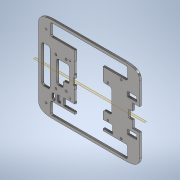
# Autodesk Inventor part: CAT_protector
Saved by Autodesk Inventor 2022 (Build 260153000, 153)
## iProperties
Created: 2024-07-28
Part Number: CAT_protector
Material: Типовые
Document SubType Name: Sheet Metal
Designer: Капустяник Андрей
Density: 1 g/cm^3
Sheet Metal Rule: По умолчанию
Appearance: Сталь — полированная
Author: Капустяник Андрей
Autodesk Inventor part; units mm, degrees
(part 1 of 2)
ref_plane "YZ Plane" through (0, 0, 0) normal (1, 0, 0) x (0, 1, 0)
ref_plane "XZ Plane" through (0, 0, 0) normal (0, 1, 0) x (-1, 0, 0)
ref_plane "XY Plane" through (0, 0, 0) normal (0, 0, 1) x (1, 0, 0)
sketch "Эскиз1" plane through (0, 0, 0) normal (0, 0, 1) x (1, 0, 0)
  line L0 (73, -60.7947) -> (73, -48.7947)
  line L1 (-3, -60.7947) -> (-73, -60.7947)
  line L2 (75, -60.7227) -> (75, -58.3095)
  line L3 (6, -60.7947) -> (70, -60.7947)
  spline S0 degree 4 poles (55, -66.7947) (62.0326, -66.7947) (73.0217, -66.3174) (75, -62.6206) (75, -58.3095) knots 0 0 0 0 0 1 1 1 1 1
  spline S1 degree 2 poles (-55, -66.7947) (-75.0547, -67.2536) (-75, -58.3095) knots 0 0 0 1 1 1
  spline S2 degree 2 poles (55, 66.7947) (75.0195, 66.261) (75, 58.3095) knots 0 0 0 1 1 1
  spline S3 degree 2 poles (-55, 66.7947) (-75.2212, 66.9636) (-75, 58.3095) knots 0 0 0 1 1 1
  line L4 (-60.2698, -62.7947) -> (55, -62.7947)
  line L5 (60, -58.3095) -> (60, -62.7947)
  line L6 (60, -62.7947) -> (55, -62.7947)
  line L7 (60, 62.7947) -> (-60, 62.7947)
  line L8 (55, 66.7947) -> (-55, 66.7947)
  line L9 (-75, 58.3095) -> (-75, -58.3095)
  line L10 (55, -66.7947) -> (-55, -66.7947)
  line L11 (75, -58.3095) -> (75, 58.3095)
  line L12 (60, -62.7947) -> (-60, -62.7947)
  line L13 (-60, 62.7947) -> (60, 62.7947)
  line L14 (-75, 40.5) -> (-75, 43.5)
  line L15 (75, 40.5) -> (75, 43.5)
  line L16 (75, -40.5) -> (75, -43.5)
  line L17 (-75, -40.5) -> (-75, -43.5)
  line L18 (-75, -40.5) -> (-75, -43.5)
  line L19 (75, -40.5) -> (75, -43.5)
  line L20 (-60, -40.5) -> (60, -40.5)
  line L21 (60, -43.5) -> (-60, -43.5)
  line L22 (-60, 43.5) -> (60, 43.5)
  line L23 (60, 40.5) -> (-60, 40.5)
  line L24 (0, -43.5) -> (4, -43.5)
  line L25 (4, -43.5) -> (4, -62.7947)
  line L26 (4, -43.5) -> (-4, -43.5)
  line L27 (-4, -43.5) -> (-4, -62.7947)
  line L28 (0, 43.5) -> (4, 43.5)
  line L29 (4, 43.5) -> (4, 62.7947)
  line L30 (4, 62.7947) -> (-4, 62.7947)
  line L31 (-4, 62.7947) -> (-4, 43.5)
  line L32 (-60, 43.5) -> (60, 43.5)
  line L33 (60, 40.5) -> (-60, 40.5)
  line L34 (-60, -43.5) -> (60, -43.5)
  line L35 (60, -40.5) -> (-60, -40.5)
  line L36 (-60, -62.7947) -> (-60, -43.5)
  line L37 (-60, -40.5) -> (-60, 40.5)
  line L38 (-60, 62.7947) -> (-60, 43.5)
  line L39 (60, 62.7947) -> (60, 43.5)
  line L40 (60, 40.5) -> (60, -40.5)
  line L41 (60, -43.5) -> (60, -58.3095)
  line L42 (60, 43.5) -> (60, -43.5)
  line L43 (-60, 43.5) -> (-60, -43.5)
  line L44 (-55, 66.7947) -> (-55, 64.6653)
  line L45 (-55, 64.6653) -> (-63.94, 64.6653)
  line L46 (-63.94, 64.6653) -> (-63.94, 58.3095)
  line L47 (-63.94, 58.3095) -> (-75, 58.3095)
  line L48 (-55, -66.7947) -> (-55, -64.5292)
  line L49 (-55, -64.5292) -> (-62.0706, -64.5292)
  line L50 (-62.0706, -64.5292) -> (-62.0706, -58.3095)
  line L51 (-62.0706, -58.3095) -> (-75, -58.3095)
  line L52 (55, -66.7947) -> (55, -65.0318)
  line L53 (55, -65.0318) -> (61.8678, -65.0318)
  line L54 (61.8678, -65.0318) -> (61.8678, -58.3095)
  line L55 (61.8678, -58.3095) -> (75, -58.3095)
  line L56 (55, 66.7947) -> (55, 64.6653)
  line L57 (55, 64.6653) -> (61.3837, 64.6653)
  line L58 (61.3837, 64.6653) -> (61.3837, 58.3095)
  line L59 (61.3837, 58.3095) -> (75, 58.3095)
  point P0 (-73, -48.7947)
  point P1 (72.3235, -63.7587)
  point P2 (-72.3272, -63.6113)
  point P3 (72.5326, 62.9869)
  point P4 (-72.4994, 63.4051)
  dimension "d14" = 4
  dimension "d15" = 8
  dimension "d16" = 4
  dimension "d17" = 8
  measures "d14" distance of L24.start L24.end
  measures "d15" distance of L24.end L26.end
  measures "d16" distance of L28.start L28.end
  measures "d17" distance of L29.end L30.end
extrude "Пластина2" add sketch "Эскиз1" along normal blind 3 contours L36 L4 L6 L5 L3 L54 L53 L52 L10 L48 L49 L50 L1 | L1 L50 L51 L9 L47 L46 L45 L44 L8 L56 L57 L58 L59 L11 L55 L54 L3 L5 L41 L42 L40 L39 L7 L38 L43 L37 L36 | L37 L23 L40 L20
sketch "Эскиз2" plane through (0, 0, 3) normal (0, 0, 1) x (1, 0, 0)
  line L0 (-75, 58.3095) -> (-75, -58.3095)
  line L1 (-75, 0) -> (-79, 0)
  line L2 (75, -58.3095) -> (75, 58.3095)
  line L3 (75, 0) -> (79, 0)
  line L4 (-79, 52.7636) -> (-79, -52.7636)
  line L5 (79, 52.7636) -> (79, -52.7636)
  line L6 (-60, 62.7947) -> (60, 62.7947)
  line L7 (60, -62.7947) -> (-60, -62.7947)
  line L8 (-75, -58.3095) -> (-75, 58.3095)
  line L9 (55, -66.7947) -> (-55, -66.7947)
  line L10 (75, 58.3095) -> (75, -58.3095)
  line L11 (-55, 66.7947) -> (55, 66.7947)
  line L12 (-55, -66.7947) -> (55, -66.7947)
  line L13 (-55, -66.7947) -> (-55, -63.9796)
  line L14 (-55, -63.9796) -> (-61.4162, -63.9796)
  line L15 (-61.4162, -63.9796) -> (-61.4162, 0)
  line L16 (-61.4162, 0) -> (-79, 0)
  line L17 (55, 66.7947) -> (-55, 66.7947)
  line L18 (-55, 66.7947) -> (-55, 63.9478)
  line L19 (-55, 63.9478) -> (-61.4162, 63.9478)
  line L20 (-61.4162, 63.9478) -> (-61.4162, 0)
  line L21 (-79, 0) -> (-61.4162, 0)
  line L22 (60, 62.7947) -> (-60, 62.7947)
  line L23 (-75, -58.3095) -> (-75, 58.3095)
  line L24 (-75, 58.3095) -> (-75, 62.3095)
  line L25 (-75, -58.3095) -> (-75, -62.3095)
  spline S0 degree 4 poles (-79, -52.7636) (-79, -59.2344) (-76.8822, -65.8429) (-63.8717, -66.7947) (-55, -66.7947) knots 0 0 0 0 0 1 1 1 1 1
  line L26 (-60, 40.5) -> (-60, 62.7947)
  line L27 (60, 62.7947) -> (60, 40.5)
  line L28 (-60, 40.5) -> (60, 40.5)
  line L29 (61.3837, 58.3095) -> (75, 58.3095)
  line L30 (61.3837, 64.6653) -> (61.3837, 58.3095)
  line L31 (55, 64.6653) -> (61.3837, 64.6653)
  line L32 (55, 66.7947) -> (55, 64.6653)
  line L33 (-55, 64.6653) -> (-55, 66.7947)
  line L34 (-63.94, 64.6653) -> (-55, 64.6653)
  line L35 (-63.94, 58.3095) -> (-63.94, 64.6653)
  line L36 (-75, 58.3095) -> (-63.94, 58.3095)
  line L37 (-62.0706, -58.3095) -> (-75, -58.3095)
  line L38 (-62.0706, -64.5292) -> (-62.0706, -58.3095)
  line L39 (-55, -64.5292) -> (-62.0706, -64.5292)
  line L40 (-55, -66.7947) -> (-55, -64.5292)
  line L41 (55, -65.0318) -> (55, -66.7947)
  line L42 (61.8678, -65.0318) -> (55, -65.0318)
  line L43 (61.8678, -58.3095) -> (61.8678, -65.0318)
  line L44 (75, -58.3095) -> (61.8678, -58.3095)
  line L45 (60, -40.5) -> (-60, -40.5)
  line L46 (60, -40.5) -> (60, -62.7947)
  line L47 (-60, -62.7947) -> (-60, -40.5)
  spline S1 degree 4 poles (-55, 66.7947) (-63.8717, 66.7947) (-76.8822, 65.8429) (-79, 59.2344) (-79, 52.7636) knots 0 0 0 0 0 1 1 1 1 1
  line L48 (-55, 66.7947) -> (55, 66.7947)
  line L49 (55, -66.7947) -> (-55, -66.7947)
  line L50 (75, -58.3095) -> (75, -62.3095)
  line L51 (75, 58.3095) -> (75, 62.3095)
  line L52 (-55, 66.7947) -> (0, 66.7947)
  line L53 (0, 66.7947) -> (55, 66.7947)
  spline S2 degree 4 poles (55, -66.7947) (63.8717, -66.7947) (76.8822, -65.8429) (79, -59.2344) (79, -52.7636) knots 0 0 0 0 0 1 1 1 1 1
  line L54 (55, 64.6653) -> (55, 66.7947)
  spline S3 degree 4 poles (55, 66.7947) (63.8717, 66.7947) (76.8822, 65.8429) (79, 59.2344) (79, 52.7636) knots 0 0 0 0 0 1 1 1 1 1
  line L55 (55, -66.7947) -> (55, -65.0318)
  line L56 (55, -65.0318) -> (60.9248, -65.0318)
  line L57 (60.9248, -65.0318) -> (60.9248, 64.6653)
  line L58 (61.3837, 64.6653) -> (55, 64.6653)
  line L59 (55, 64.6653) -> (55, 66.7947)
  line L60 (55, 64.6653) -> (60.9248, 64.6653)
  line L61 (61.8678, -65.0318) -> (55, -65.0318)
  point P0 (0, 0)
  dimension "d18" = 4
  dimension "d19" = 4
  dimension "d121" = 4
  dimension "d122" = 4
  dimension "d123" = 4
  dimension "d124" = 4
  dimension "d125" = 55
  measures "d18" distance of L1.end L1.start
  measures "d19" distance of L3.end L3.start
  measures "d121" distance of L0.start L24.end
  measures "d122" distance of L8.start L25.end
  measures "d123" distance of L10.end L50.end
  measures "d124" distance of L10.start L51.end
  measures "d125" distance of L52.end L11.end
sheet face with bend "Грань4" sketch "Эскиз2" thickness 3 toward (0, 0, -1) bend radius 3 contours L0 L1 L4 S1 L24 | L24 S1 L18 L34 L35 L36 | L0 L25 S0 L4 L1 | L37 L38 L39 L13 S0 L25 | S3 L51 L29 L30 L31 L32 | L41 L42 L43 L44 L50 S2 | S3 L5 L3 L2 L51 | L50 L2 L3 L5 S2
bend "Сгиб2"
sketch "Эскиз3" plane through (0, 0, 3) normal (0, 0, 1) x (1, 0, 0)
  line L0 (-79, 40.5) -> (-21.945, 40.5) projected
  line L1 (-62.1467, -40.5) -> (-79, -40.5) projected
  line L2 (-55, 66.7947) -> (55, 66.7947) projected
  line L3 (55, -66.7947) -> (-55, -66.7947) projected
  line L4 (60, 62.7947) -> (60, 40.5) projected
  line L5 (60, -62.7947) -> (-60, -62.7947) projected
  line L6 (-60, 40.5) -> (-60, 62.7947) projected
  line L7 (-60, 62.7947) -> (60, 62.7947) projected
  line L8 (68, -17.5) -> (79, -17.5)
  line L9 (79, -17.5) -> (79, 17.5)
  line L10 (79, 17.5) -> (68, 17.5)
  line L11 (68, 17.5) -> (68, -17.5)
  line L12 (-68, -17.5) -> (-79, -17.5) projected
  line L13 (-79, -17.5) -> (-79, -40.5) projected
  line L14 (-62.1467, -40.5) -> (-62.1467, -10.5) projected
  line L15 (-62.1467, -10.5) -> (-36.1467, -10.5) projected
  line L16 (-36.1467, -10.5) -> (-36.1467, -40.5) projected
  line L17 (-21.945, -40.5) -> (-21.945, 40.5) projected
  line L18 (-79, 40.5) -> (-79, 17.5) projected
  line L19 (-79, 17.5) -> (-68, 17.5) projected
  line L20 (-68, 17.5) -> (-68, -17.5) projected
  line L21 (-21.945, -40.5) -> (-36.1467, -40.5) projected
  line L22 (79, -5) -> (68, -5)
  line L23 (68, -5) -> (68, 5)
  line L24 (68, 5) -> (79, 5)
  line L25 (79, 5) -> (79, -5)
  line L26 (79, -5) -> (68, 5) construction
  line L27 (68, -5) -> (79, 5) construction
  line L28 (79, 52.7636) -> (79, 0) projected
  ellipse E0 centre (78.3753, -19.3) end of major axis (79, -19.3) minor radius 0.5 (78.3753, -19.8) -> (79, -19.3) ccw projected
  line L29 (79, -19.3) -> (79, -17.5) projected
  line L30 (79, -17.5) -> (68, -17.5) projected
  line L31 (68, -17.5) -> (68, -6) projected
  line L32 (68, -6) -> (63.1467, -6) projected
  arc A0 (62.1467, -5) -> (63.1467, -6) centre (63.1467, -5) ccw projected
  line L33 (62.1467, -5) -> (62.1467, 5) projected
  arc A1 (63.1467, 6) -> (62.1467, 5) centre (63.1467, 5) ccw projected
  line L34 (63.1467, 6) -> (68, 6) projected
  line L35 (68, 6) -> (68, 17.5) projected
  line L36 (68, 17.5) -> (79, 17.5) projected
  line L37 (79, 17.5) -> (79, 19.3) projected
  ellipse E1 centre (78.3753, 19.3) end of major axis (79, 19.3) minor radius 0.5 (79, 19.3) -> (78.3753, 19.8) ccw projected
  line L38 (78.3753, 19.8) -> (62.1467, 19.8) projected
  line L39 (62.1467, 19.8) -> (62.1467, 10.5) projected
  line L40 (62.1467, 10.5) -> (36.1467, 10.5) projected
  line L41 (36.1467, 10.5) -> (36.1467, 40.5) projected
  line L42 (21.945, 40.5) -> (36.1467, 40.5) projected
  line L43 (21.945, 40.5) -> (21.945, -40.5) projected
  line L44 (62.1467, -40.5) -> (21.945, -40.5) projected
  line L45 (62.1467, -40.5) -> (62.1467, -19.8) projected
  line L46 (62.1467, -19.8) -> (78.3753, -19.8) projected
  line L47 (68, -6) -> (79, -6)
  line L48 (68, 6) -> (79, 6)
  line L49 (60, -40.5) -> (-60, -40.5) projected
  line L50 (60, -40.5) -> (60, -62.7947) projected
  line L51 (-60, -62.7947) -> (-60, -40.5) projected
  line L52 (-60, 40.5) -> (60, 40.5) projected
  line L53 (-79, 52.7636) -> (-79, -52.7636) projected
  line L54 (79, -52.7636) -> (79, 52.7636) projected
  line L55 (79, -6) -> (63.1467, -6)
  line L56 (63.1467, 6) -> (79, 6)
  line L57 (79, 6) -> (79, -6)
  line L58 (68, -17.5) -> (79, -17.5)
  line L59 (79, -17.5) -> (79, 17.5)
  line L60 (79, 17.5) -> (68, 17.5)
  line L61 (68, 17.5) -> (68, -17.5)
  point P0 (0, 0)
  point P1 (79, -52.7636)
  point P2 (73.5, 0)
  dimension "d54" = 10
  constraints: 38 end point, 7 parallel, 4 collinear, 4 perpendicular, 3 horizontal, 3 point on line, 2 midpoint, 10 other
  measures "d54" distance of L22.end L23.end
extrude "Вырез1" cut sketch "Эскиз3" against normal blind 3 contours L8 L11 L47 L9 | L9 L48 L11 L10 | L47 L11 L22 L9 | L9 L24 L11 L48 | L32 A0 L33 A1 L34 L11 | L22 L11 L24 L9
sketch "Эскиз5" plane through (0, 0, 3) normal (0, 0, 1) x (1, 0, 0)
  line L0 (65.1786, -28.7) -> (72.0893, -28.7) projected
  line L1 (72.0893, -22.5) -> (65.1786, -22.5) projected
  line L2 (72.0893, 22.5) -> (65.1786, 22.5) projected
  line L3 (65.1786, 28.7) -> (72.0893, 28.7) projected
  line L4 (61.2, 28.5) -> (74.1, 28.5)
  line L5 (74.1, 28.5) -> (74.1, 22.7)
  line L6 (74.1, 22.7) -> (61.2, 22.7)
  line L7 (61.2, 22.7) -> (61.2, 28.5)
  line L8 (61.2, -22.7) -> (74.1, -22.7)
  line L9 (74.1, -22.7) -> (74.1, -28.5)
  line L10 (74.1, -28.5) -> (61.2, -28.5)
  line L11 (61.2, -28.5) -> (61.2, -22.7)
  line L12 (60.4, -21.9) -> (74.9, -21.9)
  line L13 (74.9, -21.9) -> (74.9, -29.3)
  line L14 (74.9, -29.3) -> (60.4, -29.3)
  line L15 (60.4, -29.3) -> (60.4, -21.9)
  line L16 (74.9, 29.3) -> (60.4, 29.3)
  line L17 (60.4, 29.3) -> (60.4, 21.9)
  line L18 (60.4, 21.9) -> (74.9, 21.9)
  line L19 (74.9, 21.9) -> (74.9, 29.3)
  point P0 (0, 0)
  point P1 (61.35, -39.5)
  point P2 (74.1, -27.9)
  point P3 (61.2, -22.1)
  point P4 (79, -52.7636)
  dimension "d133" = 0.8
  dimension "d134" = 0.8
  constraints: 32 end point, 8 parallel, 4 perpendicular, 2 horizontal, 13 other
  measures "d133" distance between parallel lines of L11 L15
  measures "d134" distance between parallel lines of L4 L16
extrude "Вырез3" cut sketch "Эскиз5" against normal blind 3 contours L4 L5 L6 L7 | L8 L9 L10 L11 | L12 L13 L14 L15 | L19 L18 L17 L16
sketch "Эскиз6" plane through (0, 0, 3) normal (0, 0, 1) x (1, 0, 0)
  line L0 (-22.0704, -43.5) -> (-22.0704, -28.4138)
  line L1 (-22.0704, -43.5) -> (-39.0704, -43.5)
  line L2 (-39.0704, -28.4138) -> (-39.0704, -43.5)
  line L3 (-22.0704, -28.4138) -> (-39.0704, -28.4138)
  line L4 (-60, 62.7947) -> (-60, -62.7947)
  line L5 (-22.0704, -43.5) -> (-60, -43.5)
  line L6 (-60, -43.5) -> (-60, -28.4138)
  line L7 (-60, -28.4138) -> (-22.0704, -28.4138)
  line L8 (-22.0704, -28.4138) -> (-22.0704, -43.5)
  line L9 (-22.0704, 43.5) -> (-60, 43.5)
  line L10 (-60, 43.5) -> (-60, 28.4138)
  line L11 (-60, 28.4138) -> (-22.0704, 28.4138)
  line L12 (-22.0704, 28.4138) -> (-22.0704, 43.5)
  line L13 (74.5523, 43.5) -> (-79, 43.5)
  line L14 (-68, 0) -> (-60, 0)
  line L15 (-60, 28.4138) -> (-22.0704, 28.4138)
  line L16 (-22.0704, 28.4138) -> (-32.0704, 28.4138)
  line L17 (-32.0704, 28.4138) -> (-32.0704, -28.4138)
  line L18 (-32.0704, -28.4138) -> (-22.0704, -28.4138)
  line L19 (-22.0704, -28.4138) -> (-22.0704, 28.4138)
  line L20 (-32.0704, 28.4138) -> (-60, 28.4138)
  line L21 (-60, 28.4138) -> (-60, 23.4138)
  line L22 (-60, 23.4138) -> (-32.0704, 23.4138)
  line L23 (-32.0704, 23.4138) -> (-32.0704, 28.4138)
  line L24 (-32.0704, -28.4138) -> (-60, -28.4138)
  line L25 (-60, -28.4138) -> (-60, -23.4138)
  line L26 (-60, -23.4138) -> (-32.0704, -23.4138)
  line L27 (-32.0704, -23.4138) -> (-32.0704, -28.4138)
  line L28 (-60, 23.4138) -> (-60, -23.4138)
  point P0 (0, 0)
  dimension "d45" = 10
  dimension "d52" = 5
  dimension "d53" = 5
  measures "d45" distance between parallel lines of L17 L19
  measures "d52" distance between parallel lines of L11 L22
  measures "d53" distance between parallel lines of L7 L26
sheet face with bend "Грань5" sketch "Эскиз6" thickness 3 toward (0, 0, -1) bend radius 3
bend "Сгиб3"
sketch "Эскиз7" plane through (0, 0, 3) normal (0, 0, 1) x (1, 0, 0)
  line L0 (55, -66.7947) -> (-55, -66.7947)
  line L1 (-55, 66.7947) -> (55, 66.7947)
  line L2 (-60, 43.5) -> (-60, 62.7947)
  line L3 (-60, 62.7947) -> (60, 62.7947)
  line L4 (60, 62.7947) -> (60, 40.5)
  line L5 (60, -62.7947) -> (-60, -62.7947)
  line L6 (-60, -62.7947) -> (-60, -43.5)
  spline S0 degree 4 poles (-74.5618, -40.5) (-74.5618, -41.2011) (-74.563, -41.9466) (-74.5609, -42.7177) (-74.5523, -43.5) knots 0 0 0 0 0 1 1 1 1 1
  line L7 (-74.5523, -43.5) -> (79, -43.5)
  line L8 (79, -40.5) -> (79, -43.5)
  line L9 (79, -40.5) -> (-74.5618, -40.5)
  spline S1 degree 4 poles (74.5618, 40.5) (74.5618, 41.2011) (74.563, 41.9466) (74.5609, 42.7177) (74.5523, 43.5) knots 0 0 0 0 0 1 1 1 1 1
  line L10 (74.5523, 43.5) -> (-79, 43.5)
  line L11 (-79, 40.5) -> (-79, 43.5)
  line L12 (-79, 40.5) -> (74.5618, 40.5)
  line L13 (60, -62.7947) -> (60, 62.7947)
  line L14 (60, 43.5) -> (56.75, 43.5)
  line L15 (56.75, 43.5) -> (56.75, -43.5)
  line L16 (56.75, -43.5) -> (60, -43.5)
  line L17 (60, -43.5) -> (60, 43.5)
  arc A0 (62.1467, -5) -> (63.1467, -6) centre (63.1467, -5) ccw
  line L18 (62.1467, -5) -> (62.1467, 5)
  arc A1 (63.1467, 6) -> (62.1467, 5) centre (63.1467, 5) ccw
  line L19 (-60, -43.5) -> (-22.0704, -43.5)
  line L20 (-22.0704, -43.5) -> (-22.0704, -40.5)
  line L21 (-22.0704, 43.5) -> (-60, 43.5)
  line L22 (-22.0704, 40.5) -> (60, 40.5)
  line L23 (-22.0704, 40.5) -> (-22.0704, 43.5)
  line L24 (60, -40.5) -> (-22.0704, -40.5)
  line L25 (60, -40.5) -> (60, -62.7947)
  line L26 (-79, 52.7636) -> (-79, -52.7636)
  line L27 (79, -52.7636) -> (79, -17.5)
  line L28 (79, 17.5) -> (79, 52.7636)
  line L29 (63.1467, 6) -> (68, 6)
  line L30 (68, 6) -> (68, 17.5)
  line L31 (68, 17.5) -> (79, 17.5)
  line L32 (79, -17.5) -> (68, -17.5)
  line L33 (68, -17.5) -> (68, -6)
  line L34 (68, -6) -> (63.1467, -6)
  point P0 (0, 0)
  constraints: 8 end point, 3 point on line, 2 parallel, 1 horizontal, 1 perpendicular, 8 other
sheet face with bend "Грань6" sketch "Эскиз7" thickness 3 toward (0, 0, -1) bend radius 3 contours L10 L4 L12 L15 | L12 L13 L9 L15 | L9 L13 L7 L15
bend "Сгиб4"
sketch "Эскиз8" plane through (0, 0, 3) normal (0, 0, 1) x (1, 0, 0)
  line L0 (-29.7061, 17.7) -> (-45.6809, 17.7)
  line L1 (-29.7061, -5.8) -> (-44.2713, -5.8)
  ellipse E0 centre (-48.9698, 13.2) end of major axis (-48.9698, 16.7) minor radius 1.1971 projected
  line L2 (-29.7061, 17.7) -> (-33.7061, 17.7)
  line L3 (-48.9698, 13.2) -> (-48.9698, -5.8)
  line L4 (-48.9698, -5.8) -> (-44.2713, -5.8)
  line L5 (-33.7061, 17.7) -> (-48.9698, 17.7)
  line L6 (-48.9698, 17.7) -> (-48.9698, -5.8)
  line L7 (-48.9698, -5.8) -> (-33.7061, -5.8)
  line L8 (-33.7061, -5.8) -> (-33.7061, 17.7)
  line L9 (-30.7061, 20.7) -> (-30.7061, -8.8)
  line L10 (-30.7061, -8.8) -> (-51.9698, -8.8)
  line L11 (-51.9698, -8.8) -> (-51.9698, 20.7)
  line L12 (-51.9698, 20.7) -> (-30.7061, 20.7)
  line L13 (-32.7061, 18.7) -> (-49.9698, 18.7)
  line L14 (-49.9698, 18.7) -> (-49.9698, -6.8)
  line L15 (-49.9698, -6.8) -> (-32.7061, -6.8)
  line L16 (-32.7061, -6.8) -> (-32.7061, 18.7)
  line L17 (-32.7061, 18.7) -> (-30.7061, 18.7)
  line L18 (-32.7061, -6.8) -> (-30.7061, -6.8)
  line L19 (-49.9698, 18.7) -> (-50.4698, 18.7)
  line L20 (-50.4698, 18.7) -> (-50.4698, -6.8)
  line L21 (-50.4698, -6.8) -> (-49.9698, -6.8)
  line L22 (-49.9698, -6.8) -> (-49.9698, 18.7)
  point P0 (0, 0)
  dimension "d55" = 4
  dimension "d56" = 3
  dimension "d57" = 3
  dimension "d60" = 2
  dimension "d96" = 0.5
  constraints: 46 end point, 7 perpendicular, 4 horizontal, 4 parallel, 3 point on line, 1 collinear, 1 vertical, 9 other
  measures "d55" distance of L0.start L2.end
  measures "d56" distance between parallel lines of L8 L9
  measures "d57" distance between parallel lines of L6 L11
  measures "d60" distance between parallel lines of L12 L13
  measures "d96" distance of L21.end L20.end
extrude "Вырез4" cut sketch "Эскиз8" against normal blind 3 contours L8 L1 L4 L3 E0 L6 L5 L0 | L0 L5 L6 E0 L14 L13 L16 | L0 L16 L1 L8 | L16 L17 L9 L0 | L0 L9 L1 L16 | L1 L16 L15 L14 E0 L3 L4 | L1 L9 L18 L16 | L6 L3 E0 L14 | E0 L3 L6 | L14 E0 L21 L20 L19 | L14 E0
sketch "Эскиз9" plane through (0, 0, 3) normal (0, 0, 1) x (1, 0, 0)
  line L0 (-60, 5) -> (-60, -5) projected
  line L1 (-60, 5) -> (-22.0704, 5)
  line L2 (-22.0704, 5) -> (-22.0704, -5)
  line L3 (-22.0704, -5) -> (-60, -5)
  line L4 (-60, -5) -> (-60, 5)
  line L5 (-60, -5) -> (-79, -5) projected
  line L6 (-22.0704, -5) -> (-25.0704, -5)
  line L7 (-25.0704, -5) -> (-25.0704, 5)
  line L8 (-25.0704, 5) -> (-22.0704, 5)
  line L9 (-22.0704, 5) -> (-22.0704, -5)
  line L10 (-27.1601, 11.2623) -> (-27.1601, -11.2623) projected
  line L11 (-22.0704, -43.5) -> (-22.0704, 43.5) projected
  line L12 (-22.8704, 9.6299) -> (-22.8704, 25.277) projected
  line L13 (-22.8704, -9.6299) -> (-22.8704, -25.277) projected
  line L14 (-23.1963, -10.238) -> (-23.1963, -27.6138) projected
  line L15 (-23.1963, -10.238) -> (-23.1963, -27.6138) projected
  line L16 (-23.1963, -27.6138) -> (-27.1633, -27.6138) projected
  line L17 (-23.1963, -27.6138) -> (-22.0704, -27.6138)
  line L18 (-22.0704, -27.6138) -> (-22.0704, -15.6138)
  line L19 (-22.0704, -15.6138) -> (-23.1963, -15.6138)
  line L20 (-23.1963, -15.6138) -> (-23.1963, -27.6138)
  line L21 (-23.1963, -10.238) -> (-22.0704, -10.238)
  line L22 (-22.0704, -10.238) -> (-22.0704, -22.238)
  line L23 (-22.0704, -22.238) -> (-23.1963, -22.238)
  line L24 (-23.1963, -22.238) -> (-23.1963, -10.238)
  line L25 (-23.1963, -27.6138) -> (-23.6963, -27.6138)
  line L26 (-23.6963, -27.6138) -> (-23.6963, -15.6138)
  line L27 (-23.6963, -15.6138) -> (-23.1963, -15.6138)
  line L28 (-23.1963, -15.6138) -> (-23.1963, -27.6138)
  line L29 (-23.1963, -10.238) -> (-23.6963, -10.238)
  line L30 (-23.6963, -10.238) -> (-23.6963, -22.238)
  line L31 (-23.6963, -22.238) -> (-23.1963, -22.238)
  line L32 (-23.1963, -22.238) -> (-23.1963, -10.238)
  ellipse E0 centre (-16.5786, 0) end of major axis (-16.5786, -50) minor radius 17.101 (-33.3998, 9.0085) -> (-33.3998, -9.0085) ccw projected
  ellipse E1 centre (-29.7061, 0) end of major axis (-29.7061, 13.5) minor radius 4.6173 (-27.1601, 11.2623) -> (-33.2518, 8.6474) ccw projected
  ellipse E2 centre (-29.7061, 0) end of major axis (-29.7061, 13.5) minor radius 4.6173 (-33.2518, -8.6474) -> (-27.1601, -11.2623) ccw projected
  line L33 (-33.2518, -8.6474) -> (-33.3998, -9.0085) projected
  line L34 (-33.3998, 9.0085) -> (-33.2518, 8.6474) projected
  line L35 (-22.0704, 0) -> (-23.4463, 0)
  line L36 (-23.1963, 10.238) -> (-23.1963, 27.6138)
  line L37 (-23.1963, 27.6138) -> (-22.0704, 27.6138)
  line L38 (-23.1963, 10.238) -> (-22.0704, 10.238)
  line L39 (-23.1963, 10.238) -> (-22.0704, 10.238)
  line L40 (-22.0704, 10.238) -> (-22.0704, 27.6138)
  line L41 (-22.0704, 27.6138) -> (-23.1963, 27.6138)
  line L42 (-23.1963, 27.6138) -> (-23.1963, 10.238)
  point P0 (0, 0)
  point P1 (-75, -5)
  dimension "d61" = 3
  dimension "d71" = 12
  dimension "d72" = 12
  dimension "d73" = 0.5
  constraints: 64 end point, 14 parallel, 8 horizontal, 7 perpendicular, 5 collinear, 5 symmetric about line, 3 point on line, 1 midpoint, 3 other
  measures "d61" distance of L7.end L8.end
  measures "d71" distance of L18.end L17.end
  measures "d72" distance of L21.end L22.end
  measures "d73" distance of L26.end L27.end
extrude "Вырез5" cut sketch "Эскиз9" against normal blind 3 contours L1 L2 L3 L7 | L17 L14 L23 L11 | L23 L13 L19 L11 | L19 L13 L21 L11 | L23 L14 L19 L13 | L19 L14 L21 L13 | L38 L36 L37 L11
sketch "Эскиз10" plane through (0, 0, 3) normal (0, 0, 1) x (1, 0, 0)
  line L0 (-22.0704, -35.8733) -> (-22.0704, -66.7947)
  line L1 (-19.85, -40.5) -> (74, -40.5)
  line L2 (74, 40.5) -> (-19.85, 40.5)
  line L3 (56.75, 43.5) -> (56.75, -43.5)
  line L4 (-22.0704, -43.5) -> (-22.0704, 43.5)
  line L5 (56.75, 43.5) -> (-22.0704, 43.5)
  line L6 (-22.0704, 43.5) -> (-22.0704, 40.5)
  line L7 (-22.0704, 40.5) -> (56.75, 40.5)
  line L8 (56.75, 40.5) -> (56.75, 43.5)
  line L9 (60, -43.5) -> (60, -62.7947)
  line L10 (-22.0704, -43.5) -> (-22.0704, 43.5)
  line L11 (60, -43.5) -> (-22.0704, -43.5)
  line L12 (-22.0704, -43.5) -> (-22.0704, -40.5)
  line L13 (-22.0704, -40.5) -> (60, -40.5)
  line L14 (60, -40.5) -> (60, -43.5)
  point P0 (0, 0)
  point P1 (-21.95, 40.5)
  point P2 (-22.0704, 5)
  point P3 (-22.0704, -5)
sheet face with bend "Грань7" sketch "Эскиз10" thickness 3 toward (0, 0, -1) bend radius 3 contours L13 L1 L3 L11 L0 | L4 L5 L3 L2 L7 | L3 L1 L14 L11
bend "Сгиб5"
sketch "Эскиз11" plane through (0, 0, 0) normal (0, 0, -1) x (-1, 0, 0)
  circle A0 centre (51.6714, 23.0046) radius 2.1 projected
  circle A1 centre (51.6714, -23.0046) radius 2.1 projected
  circle A2 centre (31.1704, 33.954) radius 2.1 projected
  circle A3 centre (31.1704, -33.954) radius 2.1 projected
  circle A4 centre (31.1704, -33.954) radius 2.1 projected
  circle A5 centre (31.1704, 33.954) radius 2.1 projected
  circle A6 centre (31.1704, -33.954) radius 1.5
  circle A7 centre (31.1704, 33.954) radius 1.5
  circle A8 centre (51.6714, 23.0046) radius 1.5
  circle A9 centre (51.6714, -23.0046) radius 1.5
  circle A10 centre (31.1704, -33.954) radius 2.1 projected
  line L0 (78.7, 7.7813) -> (41.2823, 7.7813) projected
  circle A11 centre (31.1704, 33.954) radius 2.1 projected
  point P0 (0, 0)
  dimension "d88" = 3
  dimension "d89" = 3
  dimension "d90" = 3
  dimension "d91" = 3
  constraints: 4 centre point, 4 coincident
  measures "d88" diameter of A6
  measures "d89" diameter of A7
  measures "d90" diameter of A8
  measures "d91" diameter of A9
extrude "Вырез6" cut sketch "Эскиз11" against normal blind 3 contours A8 | A9
fillet "Сопряжение1" radius 3 4 edges at (-30.7061, 18.7, 1.5) (-30.7061, -6.8, 1.5) (-50.4698, 18.7, 1.5) (-50.4698, -6.8, 1.5)
sketch "Эскиз13" plane through (0, 0, 3) normal (0, 0, 1) x (1, 0, 0)
  line L0 (60, 43.5) -> (-60, 43.5) projected
  line L1 (-60, 43.5) -> (-60, 62.7947) projected
  line L2 (-60, 62.7947) -> (60, 62.7947) projected
  line L3 (60, 62.7947) -> (60, 43.5) projected
  line L4 (-60, -43.5) -> (60, -43.5) projected
  line L5 (60, -43.5) -> (60, -62.7947) projected
  line L6 (60, -62.7947) -> (-60, -62.7947) projected
  line L7 (-60, -62.7947) -> (-60, -43.5) projected
  line L8 (55, -66.7947) -> (-55, -66.7947) projected
  arc A0 (62.1467, -5) -> (63.1467, -6) centre (63.1467, -5) ccw projected
  line L9 (62.1467, -5) -> (62.1467, 5) projected
  arc A1 (63.1467, 6) -> (62.1467, 5) centre (63.1467, 5) ccw projected
  line L10 (-55, 66.7947) -> (55, 66.7947) projected
  line L11 (-47.4698, 18.7) -> (-33.7061, 18.7) projected
  arc A2 (-30.7061, 15.7) -> (-33.7061, 18.7) centre (-33.7061, 15.7) ccw projected
  line L12 (-30.7061, 15.7) -> (-30.7061, -3.8) projected
  arc A3 (-33.7061, -6.8) -> (-30.7061, -3.8) centre (-33.7061, -3.8) ccw projected
  line L13 (-33.7061, -6.8) -> (-47.4698, -6.8) projected
  line L14 (-22.0704, -27.6138) -> (-23.1963, -27.6138) projected
  line L15 (-23.1963, -27.6138) -> (-23.1963, -10.238) projected
  line L16 (-23.1963, -10.238) -> (-22.0704, -10.238) projected
  line L17 (-22.0704, -5) -> (-25.0704, -5) projected
  line L18 (-25.0704, -5) -> (-25.0704, 5) projected
  line L19 (-25.0704, 5) -> (-22.0704, 5) projected
  line L20 (-22.0704, 10.238) -> (-23.1963, 10.238) projected
  line L21 (-23.1963, 10.238) -> (-23.1963, 27.6138) projected
  line L22 (-23.1963, 27.6138) -> (-22.0704, 27.6138) projected
  line L23 (-60, -43.5) -> (60, -43.5) projected
  line L24 (60, 43.5) -> (-60, 43.5) projected
  line L25 (21.945, -43.5) -> (-22.0704, -43.5)
  line L26 (-22.0704, 43.5) -> (21.945, 43.5)
  line L27 (21.945, 43.5) -> (21.945, -43.5)
  line L28 (21.945, 40.5) -> (21.945, -40.5) projected
  line L29 (-22.0704, -43.5) -> (-23.0704, -43.5)
  line L30 (-22.0704, 43.5) -> (-23.0704, 43.5)
  line L31 (-50.4698, -3.8) -> (-50.4698, 15.7) projected
  arc A4 (-47.4698, 18.7) -> (-50.4698, 15.7) centre (-47.4698, 15.7) ccw projected
  arc A5 (-50.4698, -3.8) -> (-47.4698, -6.8) centre (-47.4698, -3.8) ccw projected
  line L32 (-22.0704, 5) -> (-22.0704, -5) projected
  line L33 (-22.0704, -10.238) -> (-22.0704, -27.6138) projected
  line L34 (-22.0704, 27.6138) -> (-22.0704, 10.238) projected
  line L35 (-79, 52.7636) -> (-79, -52.7636) projected
  line L36 (79, -52.7636) -> (79, -17.5) projected
  line L37 (79, 17.5) -> (79, 52.7636) projected
  line L38 (63.1467, 6) -> (68, 6) projected
  line L39 (-21, -40.5) -> (-21, -43.5) projected
  line L40 (21, -43.5) -> (21, -40.5) projected
  line L41 (-18, 40.5) -> (-21, 40.5) projected
  line L42 (-21, 43.5) -> (-21, 40.5) projected
  line L43 (21, 40.5) -> (21, 43.5) projected
  line L44 (21, 43.5) -> (21, -43.5)
  line L45 (-60, -43.5) -> (60, -43.5) projected
  line L46 (21, 40.5) -> (21, 43.5) projected
  line L47 (-21, 43.5) -> (-21, 40.5) projected
  line L48 (-21, 43.5) -> (-22.0704, 43.5)
  line L49 (-22.0704, 43.5) -> (-22.0704, 40)
  line L50 (-21, -43.5) -> (-22.0704, -43.5)
  line L51 (-22.0704, -43.5) -> (-22.0704, -40)
  line L52 (-22.0704, -43.5) -> (-22.0704, 43.5)
  line L53 (60, 43.5) -> (-60, 43.5) projected
  line L54 (-22.0704, 40) -> (-23.0704, 40)
  line L55 (-23.0704, 40) -> (-23.0704, 43.5)
  line L56 (-23.0704, 43.5) -> (-22.0704, 43.5)
  line L57 (-22.0704, 43.5) -> (-22.0704, 40)
  line L58 (-22.0704, -40) -> (-23.0704, -40)
  line L59 (-23.0704, -40) -> (-23.0704, -43.5)
  line L60 (-23.0704, -43.5) -> (-22.0704, -43.5)
  line L61 (-22.0704, -43.5) -> (-22.0704, -40)
  line L62 (-22.0704, 27.6138) -> (-22.0704, 10.238) projected
  line L63 (21.945, -43.5) -> (-22.0704, -43.5)
  line L64 (-22.0704, -43.5) -> (-22.0704, 43.5)
  line L65 (-22.0704, 43.5) -> (21.945, 43.5)
  line L66 (21.945, 43.5) -> (21.945, -43.5)
  line L67 (68, 6) -> (68, 17.5) projected
  line L68 (68, 17.5) -> (79, 17.5) projected
  line L69 (79, -17.5) -> (68, -17.5) projected
  line L70 (68, -17.5) -> (68, -6) projected
  line L71 (68, -6) -> (63.1467, -6) projected
  point P0 (0, 0)
  dimension "d127" = 3.5
  dimension "d129" = 3.5
  dimension "d130" = 1
  dimension "d131" = 1
  constraints: 46 end point, 8 horizontal, 7 parallel, 5 perpendicular, 2 collinear, 2 point on line, 1 vertical, 13 other
  measures "d127" distance of L49.end L48.end
  measures "d129" distance of L50.end L51.end
  measures "d130" distance of L55.end L56.end
  measures "d131" distance of L60.end L59.end
extrude "Вырез7" cut sketch "Эскиз13" against normal blind 3 contours L27 L4 L40 L44 L43 L0 | L43 L44 L40 L4 L51 L52 L33 L32 L34 L49 L0
sketch "Эскиз14" plane through (0, 0, 3) normal (0, 0, 1) x (1, 0, 0)
  circle A0 centre (29.5, -25.5) radius 1.6 projected
  circle A1 centre (29.5, 25.5) radius 1.6 projected
  circle A2 centre (-29.5, 25.5) radius 1.6 projected
  circle A3 centre (-29.5, 25.5) radius 1.25
  circle A4 centre (29.5, 25.5) radius 1.25
  circle A5 centre (29.5, -25.5) radius 1.25
  circle A6 centre (-29.5, -25.5) radius 1.6 projected
  circle A7 centre (-29.5, -25.5) radius 1.25
  point P0 (-31.1704, -33.954)
  dimension "d106" = 2.5
  dimension "d107" = 2.5
  dimension "d108" = 2.5
  dimension "d110" = 2.5
  constraints: 4 centre point, 4 coincident
  measures "d106" diameter of A3
  measures "d107" diameter of A4
  measures "d108" diameter of A5
  measures "d110" diameter of A7
extrude "Вырез8" cut sketch "Эскиз14" against normal blind 3 contours A3 | A4 | A5 | A7
sketch "Эскиз18" plane through (0, 0, 3) normal (0, 0, 1) x (1, 0, 0)
  line L0 (36.945, -29.6) -> (36.945, -39.6)
  line L1 (21.945, -29.6) -> (36.945, -29.6)
  line L2 (36.945, -39.6) -> (31.5198, -39.6)
  line L3 (-50.4698, -3.8) -> (-50.4698, 15.7)
  arc A0 (-47.4698, 18.7) -> (-50.4698, 15.7) centre (-47.4698, 15.7) ccw
  line L4 (-47.4698, 18.7) -> (-33.7061, 18.7)
  arc A1 (-30.7061, 15.7) -> (-33.7061, 18.7) centre (-33.7061, 15.7) ccw
  line L5 (-30.7061, 15.7) -> (-30.7061, -3.8)
  arc A2 (-33.7061, -6.8) -> (-30.7061, -3.8) centre (-33.7061, -3.8) ccw
  line L6 (-33.7061, -6.8) -> (-47.4698, -6.8)
  arc A3 (-50.4698, -3.8) -> (-47.4698, -6.8) centre (-47.4698, -3.8) ccw
  circle A4 centre (-51.6714, -23.0046) radius 1.5
  circle A5 centre (-51.6714, 23.0046) radius 1.5
  line L7 (60, 43.5) -> (21.945, 43.5)
  line L8 (-60, 43.5) -> (-60, 62.7947)
  line L9 (-60, 62.7947) -> (60, 62.7947)
  line L10 (60, 62.7947) -> (60, 43.5)
  line L11 (60, -43.5) -> (60, -62.7947)
  line L12 (60, -62.7947) -> (-60, -62.7947)
  line L13 (-60, -62.7947) -> (-60, -43.5)
  line L14 (-22.0704, -27.6138) -> (-23.1963, -27.6138)
  line L15 (-23.1963, -27.6138) -> (-23.1963, -10.238)
  line L16 (-23.1963, -10.238) -> (-22.0704, -10.238)
  line L17 (-22.0704, -5) -> (-25.0704, -5)
  line L18 (-25.0704, -5) -> (-25.0704, 5)
  line L19 (-25.0704, 5) -> (-22.0704, 5)
  line L20 (-22.0704, 10.238) -> (-23.1963, 10.238)
  line L21 (-23.1963, 10.238) -> (-23.1963, 27.6138)
  line L22 (-23.1963, 27.6138) -> (-22.0704, 27.6138)
  circle A6 centre (-29.5, -25.5) radius 1.25
  circle A7 centre (29.5, 25.5) radius 1.25
  circle A8 centre (29.5, -25.5) radius 1.25
  circle A9 centre (-29.5, 25.5) radius 1.25
  line L23 (-55, 66.7947) -> (55, 66.7947)
  line L24 (55, -66.7947) -> (-55, -66.7947)
  arc A10 (62.1467, -5) -> (63.1467, -6) centre (63.1467, -5) ccw
  line L25 (62.1467, -5) -> (62.1467, 5)
  arc A11 (63.1467, 6) -> (62.1467, 5) centre (63.1467, 5) ccw
  line L26 (-22.7204, -40.6) -> (-39.6204, -40.6)
  line L27 (-23.7204, -29.6) -> (-37.9129, -29.6)
  line L28 (-22.7204, -29.6) -> (-39.6204, -29.6)
  line L29 (-39.6204, -29.6) -> (36.945, -29.6)
  line L30 (36.945, -39.6) -> (-39.6204, -39.6)
  line L31 (-39.6204, -39.6) -> (-39.6204, -40.6)
  line L32 (-39.6204, -40.6) -> (36.945, -40.6)
  line L33 (36.945, -40.6) -> (36.945, -39.6)
  line L34 (-39.6204, -29.6) -> (-39.6204, -39.6)
  line L35 (21.945, -29.6) -> (36.945, -29.6)
  line L36 (36.945, -29.6) -> (36.945, -28.1)
  line L37 (36.945, -28.1) -> (21.945, -28.1)
  line L38 (21.945, -28.1) -> (21.945, -29.6)
  line L39 (-79, 52.7636) -> (-79, -52.7636)
  line L40 (79, -52.7636) -> (79, -17.5)
  line L41 (79, 17.5) -> (79, 52.7636)
  line L42 (63.1467, 6) -> (68, 6)
  line L43 (-60, -43.5) -> (-22.0704, -43.5)
  line L44 (-22.0704, -10.238) -> (-22.0704, -5)
  line L45 (-22.0704, 5) -> (-22.0704, 10.238)
  line L46 (-22.0704, 27.6138) -> (-22.0704, 43.5)
  line L47 (-22.0704, 43.5) -> (-60, 43.5)
  line L48 (21.945, 43.5) -> (21.945, -43.5)
  line L49 (21.945, -43.5) -> (60, -43.5)
  line L50 (-22.0704, -43.5) -> (-22.0704, -27.6138)
  line L51 (68, 6) -> (68, 17.5)
  line L52 (68, 17.5) -> (79, 17.5)
  line L53 (79, -17.5) -> (68, -17.5)
  line L54 (68, -17.5) -> (68, -6)
  line L55 (68, -6) -> (63.1467, -6)
  point P0 (0, 0)
extrude "Вырез11" cut sketch "Эскиз18" against normal blind 3 contours L0 L2 L30 L48 L1 | L1 L38 L37 L36 | L33 L32 L48 L30 L2 | L48 L30 L50 L29 | L50 L30 L34 L28 L27 L29 | L48 L32 L50 L30 | L50 L32 L26 L31 L30
sketch "Эскиз19" plane through (0, 0, 3) normal (0, 0, 1) x (1, 0, 0)
  line L0 (32.4467, -6.7) -> (32.4467, 13.7)
  line L1 (32.4467, 13.7) -> (28.4467, 13.7)
  line L2 (28.4467, 13.7) -> (28.4467, -6.7)
  line L3 (28.4467, -6.7) -> (32.4467, -6.7)
  circle A0 centre (27.9467, 17.5) radius 1.6
  circle A1 centre (27.9467, -10.5) radius 1.6
  spline S0 degree 3 poles (63.6588, 29) (63.7235, 29) (63.7997, 29.0148) (63.9185, 29.063) (63.9826, 29.1046) (64.0726, 29.1925) (64.1149, 29.254) (64.1629, 29.3674) (64.1776, 29.439) (64.1776, 29.5) knots 0 0 0 0 0.25714 0.25714 0.510158 0.510158 0.757535 0.757535 1 1 1 1
  line L4 (60.1467, 29) -> (63.6588, 29)
  arc A2 (60.1467, 29) -> (59.1467, 28) centre (60.1467, 28) ccw
  line L5 (59.1467, 23.2) -> (59.1467, 28)
  arc A3 (59.1467, 23.2) -> (60.1467, 22.2) centre (60.1467, 23.2) ccw
  line L6 (67, 22.2) -> (60.1467, 22.2)
  arc A4 (68, 21.2) -> (67, 22.2) centre (67, 21.2) ccw
  line L7 (68, 6) -> (68, 21.2)
  line L8 (63.1467, 6) -> (68, 6)
  arc A5 (63.1467, 6) -> (62.1467, 5) centre (63.1467, 5) ccw
  line L9 (62.1467, -5) -> (62.1467, 5)
  arc A6 (62.1467, -5) -> (63.1467, -6) centre (63.1467, -5) ccw
  line L10 (68, -6) -> (63.1467, -6)
  line L11 (68, -14) -> (68, -6)
  line L12 (26.1467, -14) -> (68, -14)
  arc A7 (24.4467, -12.3) -> (26.1467, -14) centre (26.1467, -12.3) ccw
  line L13 (24.4467, 19.3) -> (24.4467, -12.3)
  arc A8 (26.1467, 21) -> (24.4467, 19.3) centre (26.1467, 19.3) ccw
  line L14 (34.1467, 21) -> (26.1467, 21)
  arc A9 (34.1467, 21) -> (36.4467, 23.3) centre (34.1467, 23.3) ccw
  line L15 (36.4467, 29.7) -> (36.4467, 23.3)
  arc A10 (36.4467, 29.7) -> (34.1467, 32) centre (34.1467, 29.7) ccw
  line L16 (32.1967, 32) -> (34.1467, 32)
  arc A11 (32.1967, 40.5) -> (32.1967, 32) centre (32.1967, 36.25) ccw
  line L17 (66.0967, 40.5) -> (32.1967, 40.5)
  arc A12 (66.0967, 32) -> (66.0967, 40.5) centre (66.0967, 36.25) ccw
  line L18 (64.6989, 32) -> (66.0967, 32)
  spline S1 degree 3 poles (64.1776, 31.5) (64.1776, 31.5609) (64.1923, 31.6325) (64.2403, 31.7458) (64.2825, 31.8072) (64.3726, 31.8952) (64.4369, 31.9368) (64.5566, 31.9852) (64.6336, 32) (64.6989, 32) knots 0 0 0 0 0.241518 0.241518 0.487947 0.487947 0.74085 0.74085 1 1 1 1
  line L19 (64.1776, 29.5) -> (64.1776, 31.5)
  circle A13 centre (66.0967, 36.25) radius 1.6
  circle A14 centre (32.1967, 36.25) radius 1.6
  line L20 (25.4467, 16.7) -> (35.4467, 16.7)
  line L21 (35.4467, 16.7) -> (35.4467, -9.7)
  line L22 (35.4467, -9.7) -> (25.4467, -9.7)
  line L23 (25.4467, -9.7) -> (25.4467, 16.7)
  circle A15 centre (27.9467, -10.5) radius 4.6
  circle A16 centre (27.9467, 17.5) radius 4.6
  line L24 (35.4467, -15.1) -> (21.945, -15.1)
  line L25 (21.945, -15.1) -> (21.945, 22.1)
  line L26 (21.945, 22.1) -> (35.4467, 22.1)
  line L27 (35.4467, 22.1) -> (35.4467, -15.1)
  line L28 (21.945, 43.5) -> (21.945, -28.1)
  point P0 (0, 0)
  dimension "d135" = 3
  dimension "d136" = 3
  dimension "d137" = 3
  constraints: 16 end point, 2 centre point, 2 collinear, 2 parallel, 2 tangent, 1 horizontal, 1 perpendicular, 3 other
  measures "d135" distance between parallel lines of L1 L20
  measures "d136" radial gap between concentric circles of A1 A15
  measures "d137" radial gap between concentric circles of A0 A16
extrude "Вырез12" cut sketch "Эскиз19" against normal blind 3 contours L3 A15 L2 A16 L1 L0 | L0 L1 A16 L20 L21 L22 A15 L3 | A15 L22 A1 L23 L2 L3 | L3 L2 A15 | A16 L2 L1 | L1 L2 A16 L23 L20 A0 | A15 L12 A7 L13 L23 L22 A1 | L22 L27 L12 A15 | A15 L23 A16 L2 | A16 L14 A9 L27 L20 | L20 A0 L23 A16 L13 A8 L14 | L22 A1 | A1 L22 | A15 L13 A16 L23 | L20 A0 | A0 L20 | L27 L24 A15 L12 | A15 L13 A7 L12 | A15 L24 L25 L26 A16 L13 | A16 L14 A8 L13 | A9 L14 A16 L26 L27
fillet "Сопряжение3" radius 3 4 edges at (35.4467, -15.1, 1.5) (21.945, -15.1, 1.5) (35.4467, 22.1, 1.5) (21.945, 22.1, 1.5)
fillet "Сопряжение4" radius 2 8 edges at (-60, -43.5, 1.5) (-60, -62.7947, 1.5) (60, -43.5, 1.5) (60, -62.7947, 1.5) (60, 62.7947, 1.5) (60, 43.5, 1.5) (-60, 62.7947, 1.5) (-60, 43.5, 1.5)
ref_plane "РабПлоскость1" through (63.1467, 0, 3) normal (0, 1, 0) x (1, 0, 0)
sketch "Эскиз20" plane through (0, 0, 0) normal (0, 0, -1) x (-1, 0, 0)
  arc A0 (-24.945, 22.1) -> (-21.945, 25.1) centre (-24.945, 25.1) ccw projected
  line L0 (-21.945, 25.1) -> (-21.945, 43.5) projected
  line L1 (-58, 43.5) -> (-21.945, 43.5) projected
  arc A1 (-60, 45.5) -> (-58, 43.5) centre (-58, 45.5) ccw projected
  line L2 (-60, 45.5) -> (-60, 60.7947) projected
  arc A2 (-58, 62.7947) -> (-60, 60.7947) centre (-58, 60.7947) ccw projected
  line L3 (-58, 62.7947) -> (58, 62.7947) projected
  arc A3 (60, 60.7947) -> (58, 62.7947) centre (58, 60.7947) ccw projected
  line L4 (60, 60.7947) -> (60, 45.5) projected
  arc A4 (58, 43.5) -> (60, 45.5) centre (58, 45.5) ccw projected
  line L5 (22.0704, 43.5) -> (58, 43.5) projected
  line L6 (22.0704, 43.5) -> (22.0704, 27.6138) projected
  line L7 (22.0704, 27.6138) -> (23.1963, 27.6138) projected
  line L8 (23.1963, 27.6138) -> (23.1963, 10.238) projected
  line L9 (23.1963, 10.238) -> (22.0704, 10.238) projected
  line L10 (22.0704, 10.238) -> (22.0704, 5) projected
  line L11 (22.0704, 5) -> (25.0704, 5) projected
  line L12 (25.0704, 5) -> (25.0704, -5) projected
  line L13 (25.0704, -5) -> (22.0704, -5) projected
  line L14 (22.0704, -5) -> (22.0704, -10.238) projected
  line L15 (22.0704, -10.238) -> (23.1963, -10.238) projected
  line L16 (23.1963, -10.238) -> (23.1963, -27.6138) projected
  line L17 (23.1963, -27.6138) -> (22.0704, -27.6138) projected
  line L18 (22.0704, -27.6138) -> (22.0704, -29.6) projected
  line L19 (22.0704, -29.6) -> (39.6204, -29.6) projected
  line L20 (39.6204, -29.6) -> (39.6204, -40.6) projected
  line L21 (39.6204, -40.6) -> (22.0704, -40.6) projected
  line L22 (22.0704, -40.6) -> (22.0704, -43.5) projected
  line L23 (58, -43.5) -> (22.0704, -43.5) projected
  arc A5 (60, -45.5) -> (58, -43.5) centre (58, -45.5) ccw projected
  line L24 (60, -45.5) -> (60, -60.7947) projected
  arc A6 (58, -62.7947) -> (60, -60.7947) centre (58, -60.7947) ccw projected
  line L25 (58, -62.7947) -> (-58, -62.7947) projected
  arc A7 (-60, -60.7947) -> (-58, -62.7947) centre (-58, -60.7947) ccw projected
  line L26 (-60, -60.7947) -> (-60, -45.5) projected
  arc A8 (-58, -43.5) -> (-60, -45.5) centre (-58, -45.5) ccw projected
  line L27 (-21.945, -43.5) -> (-58, -43.5) projected
  line L28 (-21.945, -43.5) -> (-21.945, -40.6) projected
  line L29 (-21.945, -40.6) -> (-36.945, -40.6) projected
  line L30 (-36.945, -40.6) -> (-36.945, -28.1) projected
  line L31 (-36.945, -28.1) -> (-21.945, -28.1) projected
  line L32 (-21.945, -28.1) -> (-21.945, -18.1) projected
  arc A9 (-21.945, -18.1) -> (-24.945, -15.1) centre (-24.945, -18.1) ccw projected
  line L33 (-24.945, -15.1) -> (-32.4467, -15.1) projected
  arc A10 (-35.4467, -12.1) -> (-32.4467, -15.1) centre (-32.4467, -12.1) ccw projected
  line L34 (-35.4467, -12.1) -> (-35.4467, 19.1) projected
  arc A11 (-32.4467, 22.1) -> (-35.4467, 19.1) centre (-32.4467, 19.1) ccw projected
  line L35 (-32.4467, 22.1) -> (-24.945, 22.1) projected
  circle A12 centre (29.5, 25.5) radius 1.25 projected
  circle A13 centre (-29.5, -25.5) radius 1.25 projected
  circle A14 centre (-29.5, 25.5) radius 1.25 projected
  circle A15 centre (29.5, -25.5) radius 1.25 projected
  line L36 (50.4698, 15.7) -> (50.4698, -3.8) projected
  arc A16 (47.4698, -6.8) -> (50.4698, -3.8) centre (47.4698, -3.8) ccw projected
  line L37 (47.4698, -6.8) -> (33.7061, -6.8) projected
  arc A17 (30.7061, -3.8) -> (33.7061, -6.8) centre (33.7061, -3.8) ccw projected
  line L38 (30.7061, -3.8) -> (30.7061, 15.7) projected
  arc A18 (33.7061, 18.7) -> (30.7061, 15.7) centre (33.7061, 15.7) ccw projected
  line L39 (33.7061, 18.7) -> (47.4698, 18.7) projected
  arc A19 (50.4698, 15.7) -> (47.4698, 18.7) centre (47.4698, 15.7) ccw projected
  line L40 (-68, -17.5) -> (-79, -17.5) projected
  line L41 (-79, -52.7636) -> (-79, -17.5) projected
  line L42 (55, -66.7947) -> (-55, -66.7947) projected
  line L43 (79, 52.7636) -> (79, -52.7636) projected
  line L44 (-55, 66.7947) -> (55, 66.7947) projected
  line L45 (-79, 17.5) -> (-79, 52.7636) projected
  line L46 (-79, 17.5) -> (-68, 17.5) projected
  line L47 (-68, 17.5) -> (-68, 6) projected
  line L48 (-68, 6) -> (-63.1467, 6) projected
  arc A20 (-62.1467, 5) -> (-63.1467, 6) centre (-63.1467, 5) ccw projected
  line L49 (-62.1467, 5) -> (-62.1467, -5) projected
  arc A21 (-63.1467, -6) -> (-62.1467, -5) centre (-63.1467, -5) ccw projected
  line L50 (-63.1467, -6) -> (-68, -6) projected
  line L51 (-68, -6) -> (-68, -17.5) projected
  line L52 (-60.4, 29.3) -> (-60.4, 21.9) projected
  line L53 (-60.4, 21.9) -> (-74.9, 21.9) projected
  line L54 (-74.9, 21.9) -> (-74.9, 29.3) projected
  line L55 (-74.9, 29.3) -> (-60.4, 29.3) projected
  line L56 (-60.4, -21.9) -> (-60.4, -29.3) projected
  line L57 (-60.4, -29.3) -> (-74.9, -29.3) projected
  line L58 (-74.9, -29.3) -> (-74.9, -21.9) projected
  line L59 (-74.9, -21.9) -> (-60.4, -21.9) projected
  circle A22 centre (51.6714, -23.0046) radius 1.5 projected
  circle A23 centre (51.6714, 23.0046) radius 1.5 projected
  arc A24 (47.4698, -6.8) -> (50.4698, -3.8) centre (47.4698, -3.8) ccw projected
  line L60 (50.4698, -3.8) -> (40.4698, -3.8)
  line L61 (40.4698, -3.8) -> (40.4698, -16.8)
  line L62 (40.4698, -16.8) -> (50.4698, -16.8)
  line L63 (50.4698, -16.8) -> (50.4698, -3.8)
  point P0 (0, 0)
  dimension "d142" = 13
  dimension "d143" = 10
  constraints: 8 end point, 2 parallel, 1 horizontal, 1 perpendicular, 8 other
  measures "d142" distance between parallel lines of L62 L60
  measures "d143" distance between parallel lines of L63 L61
extrude "Вырез13" cut sketch "Эскиз20" against normal blind 3 contours L63 L62 L61 L37 A16 | A16 L37 L61 L60
fillet "Сопряжение5" radius 2 3 edges at (-40.4698, -6.8, 1.5) (-40.4698, -16.8, 1.5) (-50.4698, -16.8, 1.5)
sketch "Эскиз21" plane through (0, 0, 3) normal (0, 0, 1) x (1, 0, 0)
  line L0 (-79, -28.1138) -> (-39.9204, -28.1138) projected
  circle A0 centre (-29.5, 25.5) radius 1.25 projected
  circle A1 centre (29.5, -25.5) radius 1.25 projected
  circle A2 centre (29.5, 25.5) radius 1.25 projected
  circle A3 centre (-29.5, -25.5) radius 1.25 projected
  line L1 (79, -17.5) -> (68, -17.5) projected
  line L2 (68, -17.5) -> (68, -6) projected
  line L3 (68, -6) -> (63.1467, -6) projected
  arc A4 (62.1467, -5) -> (63.1467, -6) centre (63.1467, -5) ccw projected
  line L4 (62.1467, -5) -> (62.1467, 5) projected
  arc A5 (63.1467, 6) -> (62.1467, 5) centre (63.1467, 5) ccw projected
  line L5 (63.1467, 6) -> (68, 6) projected
  line L6 (68, 6) -> (68, 17.5) projected
  line L7 (68, 17.5) -> (79, 17.5) projected
  line L8 (79, 17.5) -> (79, 52.7636) projected
  line L9 (-55, 66.7947) -> (55, 66.7947) projected
  line L10 (-79, 52.7636) -> (-79, -52.7636) projected
  line L11 (55, -66.7947) -> (-55, -66.7947) projected
  line L12 (79, -52.7636) -> (79, -17.5) projected
  line L13 (60.4, 21.9) -> (60.4, 29.3) projected
  line L14 (60.4, 29.3) -> (74.9, 29.3) projected
  line L15 (74.9, 29.3) -> (74.9, 21.9) projected
  line L16 (74.9, 21.9) -> (60.4, 21.9) projected
  line L17 (60.4, -29.3) -> (60.4, -21.9) projected
  line L18 (60.4, -21.9) -> (74.9, -21.9) projected
  line L19 (74.9, -21.9) -> (74.9, -29.3) projected
  line L20 (74.9, -29.3) -> (60.4, -29.3) projected
  circle A6 centre (-51.6714, -23.0046) radius 1.5 projected
  circle A7 centre (-51.6714, 23.0046) radius 1.5 projected
  arc A8 (21.945, 25.1) -> (24.945, 22.1) centre (24.945, 25.1) ccw projected
  line L21 (24.945, 22.1) -> (32.4467, 22.1) projected
  arc A9 (35.4467, 19.1) -> (32.4467, 22.1) centre (32.4467, 19.1) ccw projected
  line L22 (35.4467, 19.1) -> (35.4467, -12.1) projected
  arc A10 (32.4467, -15.1) -> (35.4467, -12.1) centre (32.4467, -12.1) ccw projected
  line L23 (32.4467, -15.1) -> (24.945, -15.1) projected
  arc A11 (24.945, -15.1) -> (21.945, -18.1) centre (24.945, -18.1) ccw projected
  line L24 (21.945, -18.1) -> (21.945, -28.1) projected
  line L25 (21.945, -28.1) -> (36.945, -28.1) projected
  line L26 (36.945, -28.1) -> (36.945, -40.6) projected
  line L27 (36.945, -40.6) -> (21.945, -40.6) projected
  line L28 (21.945, -40.6) -> (21.945, -43.5) projected
  line L29 (21.945, -43.5) -> (58, -43.5) projected
  arc A12 (60, -45.5) -> (58, -43.5) centre (58, -45.5) ccw projected
  line L30 (60, -45.5) -> (60, -60.7947) projected
  arc A13 (58, -62.7947) -> (60, -60.7947) centre (58, -60.7947) ccw projected
  line L31 (58, -62.7947) -> (-58, -62.7947) projected
  arc A14 (-60, -60.7947) -> (-58, -62.7947) centre (-58, -60.7947) ccw projected
  line L32 (-60, -60.7947) -> (-60, -45.5) projected
  arc A15 (-58, -43.5) -> (-60, -45.5) centre (-58, -45.5) ccw projected
  line L33 (-58, -43.5) -> (-22.0704, -43.5) projected
  line L34 (-22.0704, -43.5) -> (-22.0704, -40.6) projected
  line L35 (-22.0704, -40.6) -> (-39.6204, -40.6) projected
  line L36 (-39.6204, -40.6) -> (-39.6204, -29.6) projected
  line L37 (-39.6204, -29.6) -> (-22.0704, -29.6) projected
  line L38 (-22.0704, -29.6) -> (-22.0704, -27.6138) projected
  line L39 (-22.0704, -27.6138) -> (-23.1963, -27.6138) projected
  line L40 (-23.1963, -27.6138) -> (-23.1963, -10.238) projected
  line L41 (-23.1963, -10.238) -> (-22.0704, -10.238) projected
  line L42 (-22.0704, -10.238) -> (-22.0704, -5) projected
  line L43 (-22.0704, -5) -> (-25.0704, -5) projected
  line L44 (-25.0704, -5) -> (-25.0704, 5) projected
  line L45 (-25.0704, 5) -> (-22.0704, 5) projected
  line L46 (-22.0704, 5) -> (-22.0704, 10.238) projected
  line L47 (-22.0704, 10.238) -> (-23.1963, 10.238) projected
  line L48 (-23.1963, 10.238) -> (-23.1963, 27.6138) projected
  line L49 (-23.1963, 27.6138) -> (-22.0704, 27.6138) projected
  line L50 (-22.0704, 27.6138) -> (-22.0704, 43.5) projected
  line L51 (-22.0704, 43.5) -> (-58, 43.5) projected
  arc A16 (-60, 45.5) -> (-58, 43.5) centre (-58, 45.5) ccw projected
  line L52 (-60, 45.5) -> (-60, 60.7947) projected
  arc A17 (-58, 62.7947) -> (-60, 60.7947) centre (-58, 60.7947) ccw projected
  line L53 (-58, 62.7947) -> (58, 62.7947) projected
  arc A18 (60, 60.7947) -> (58, 62.7947) centre (58, 60.7947) ccw projected
  line L54 (60, 60.7947) -> (60, 45.5) projected
  arc A19 (58, 43.5) -> (60, 45.5) centre (58, 45.5) ccw projected
  line L55 (58, 43.5) -> (21.945, 43.5) projected
  line L56 (21.945, 43.5) -> (21.945, 25.1) projected
  arc A20 (-38.4698, -6.8) -> (-40.4698, -8.8) centre (-38.4698, -8.8) ccw projected
  line L57 (-40.4698, -8.8) -> (-40.4698, -14.8) projected
  arc A21 (-42.4698, -16.8) -> (-40.4698, -14.8) centre (-42.4698, -14.8) ccw projected
  line L58 (-42.4698, -16.8) -> (-48.4698, -16.8) projected
  arc A22 (-50.4698, -14.8) -> (-48.4698, -16.8) centre (-48.4698, -14.8) ccw projected
  line L59 (-50.4698, -14.8) -> (-50.4698, 15.7) projected
  arc A23 (-47.4698, 18.7) -> (-50.4698, 15.7) centre (-47.4698, 15.7) ccw projected
  line L60 (-47.4698, 18.7) -> (-33.7061, 18.7) projected
  arc A24 (-30.7061, 15.7) -> (-33.7061, 18.7) centre (-33.7061, 15.7) ccw projected
  line L61 (-30.7061, 15.7) -> (-30.7061, -3.8) projected
  arc A25 (-33.7061, -6.8) -> (-30.7061, -3.8) centre (-33.7061, -3.8) ccw projected
  line L62 (-33.7061, -6.8) -> (-38.4698, -6.8) projected
  line L63 (-60, -66.6543) -> (-60, -28.4138) projected
  line L64 (-48.4698, -31.1) -> (-45.4698, -31.1)
  line L65 (-45.4698, -31.1) -> (-45.4698, -39.1)
  line L66 (-45.4698, -39.1) -> (-48.4698, -39.1)
  line L67 (-48.4698, -39.1) -> (-48.4698, -31.1)
  line L68 (-49.4698, -40.1) -> (-44.4698, -40.1)
  line L69 (-44.4698, -40.1) -> (-44.4698, -30.1)
  line L70 (-44.4698, -30.1) -> (-49.4698, -30.1)
  line L71 (-49.4698, -30.1) -> (-49.4698, -40.1)
  line L72 (-39.6204, -29.6) -> (-39.6204, -40.6) projected
  line L73 (-39.6204, -40.6) -> (-39.6204, -29.6) projected
  line L74 (-42.4698, -16.8) -> (-48.4698, -16.8) projected
  line L75 (-49.4698, -35.1) -> (-44.4698, -35.1)
  point P0 (0, 0)
  point P1 (-45.4698, -16.8)
  point P2 (-45.4698, -16.8)
  point P3 (-39.6204, -35.1)
  dimension "d147" = 3
  dimension "d148" = 8
  dimension "d149" = 1
  constraints: 18 end point, 5 midpoint, 4 parallel, 2 perpendicular, 2 point on line, 1 horizontal, 11 other
  measures "d147" distance of L65.end L66.end
  measures "d148" distance of L64.end L65.end
  measures "d149" distance between parallel lines of L66 L68
extrude "Вырез14" cut sketch "Эскиз21" against normal blind 3 contours L67 L75 L71 L70 L69 L65 L64 | L64 L65 L75 L67 | L75 L65 L66 L67 | L67 L66 L65 L75 L69 L68 L71
fillet "Сопряжение6" radius 1 4 edges at (-49.4698, -30.1, 1.5) (-44.4698, -30.1, 1.5) (-44.4698, -40.1, 1.5) (-49.4698, -40.1, 1.5)